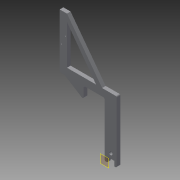
# Autodesk Inventor part: Right Climber Hook
Saved by Autodesk Inventor 2013 (Build 170138000, 138)
## iProperties
Created: 2013-03-16
Part Number: Right Climber Hook
Material: Generic
Document SubType Name: Modeling
Designer: Arpan
Density: 1 g/cm^3
Author: Arpan
Autodesk Inventor part; units mm, degrees
ref_plane "YZ Plane" through (0, 0, 0) normal (1, 0, 0) x (0, 1, 0)
ref_plane "XZ Plane" through (0, 0, 0) normal (0, 1, 0) x (-1, 0, 0)
ref_plane "XY Plane" through (0, 0, 0) normal (0, 0, 1) x (1, 0, 0)
ref_plane "Work Plane1" through (0, 0, 9.525) normal (0, 0, 1) x (1, 0, 0)
sketch "Sketch1" plane through (0, 0, 0) normal (0, 0, 1) x (1, 0, 0)
  line L0 (0, 0) -> (6.35, 0)
  line L1 (6.35, 0) -> (6.35, 12.7)
  line L2 (6.35, 12.7) -> (25.4, 12.7)
  line L3 (25.4, 12.7) -> (25.4, 0)
  line L4 (25.4, 0) -> (31.75, 0)
  line L5 (31.75, 0) -> (31.75, 161.925)
  circle A0 centre (15.875, 25.4) radius 4.7816
  line L6 (-117.475, 161.925) -> (-117.475, 142.875)
  line L7 (0, 142.875) -> (0, 0)
  line L8 (-117.475, 142.875) -> (-117.475, 284.6917)
  line L9 (-54.61, 142.875) -> (-54.61, 111.125)
  line L10 (-54.61, 111.125) -> (-105.41, 142.875)
  line L11 (-117.475, 142.875) -> (-105.41, 142.875)
  line L12 (-54.61, 142.875) -> (0, 142.875)
  line L13 (-98.425, 284.6917) -> (-117.475, 284.6917)
  line L14 (-98.425, 265.5175) -> (-98.425, 256.0855)
  line L15 (-98.425, 238.125) -> (-98.425, 161.925)
  line L16 (31.75, 161.925) -> (-6.4592, 161.925)
  line L17 (-22.225, 161.925) -> (-98.425, 161.925)
  line L18 (-98.425, 284.6917) -> (-6.4592, 161.925)
  line L19 (-22.225, 161.925) -> (-98.425, 265.5175)
  line L20 (-98.425, 238.125) -> (-98.425, 256.0855)
  point P0 (-98.425, 263.525)
  point P1 (-6.35, 161.925)
  dimension "d0" = 6.35
  dimension "d1" = 12.7
  dimension "d2" = 19.05
  dimension "d3" = 6.35
  dimension "d4" = 161.925
  dimension "d5" = 9.5631
  dimension "d6" = 12.7
  dimension "d7" = 9.525
  dimension "d8" = 149.225
  dimension "d9" = 19.05
  dimension "d12" = 54.61
  dimension "d13" = 31.75
  dimension "d14" = 50.8
  dimension "d18" = 127
  dimension "d34" = 122.7667
  dimension "d37" = 19.05
  dimension "d38" = 19.05
  dimension "d39" = 76.2
  dimension "d40" = 76.2
  dimension "d41" = 19.05
  dimension "d50" = 0.5
  dimension "d51" = 12.7
  constraints: 42 end point, 15 perpendicular, 5 parallel, 3 horizontal, 1 centre point, 1 point on line, 1 vertical
  measures "d0" distance of L0.start L0.end
  measures "d1" distance of L0.end L1.end
  measures "d2" distance of L1.end L2.end
  measures "d3" distance of L3.end L4.end
  measures "d4" distance of L4.end L5.end
  measures "d5" diameter of A0
  measures "d6" distance from line of L2 A0.centre
  measures "d7" distance from line of L1 A0.centre
  measures "d8" distance of L5.end L6.start
  measures "d9" distance of L6.start L6.end
  measures "d12" distance between parallel lines of L7 L9
  measures "d13" distance of L9.start L9.end
  measures "d14" distance from line of L9 L10.end
  measures "d18" distance of L17.start point (-98.425, 263.525)
  measures "d34" distance of L15.end L13.start
  measures "d37" distance between parallel lines of L17 L12
  measures "d38" distance between parallel lines of L8 L15
  measures "d39" distance from line of L17 L15.start
  measures "d40" distance from line of L17.start L15
  measures "d41" distance of L13.start L8.end
  measures "d50" angle of L18 L19
  measures "d51" distance from line of L16.end L19
sketch "Sketch2" plane through (0, 0, 9.525) normal (0, 0, 1) x (1, 0, 0)
  line L0 (-98.425, 298.45) -> (-117.475, 298.45) projected
  line L1 (-117.475, 284.6917) -> (-117.475, 142.875) projected
  circle A0 centre (-102.9208, 232.0925) radius 1.5875
  circle A1 centre (-113.03, 209.0801) radius 1.5875
  dimension "d24" = 3.175
  dimension "d25" = 14.5542
  dimension "d26" = 66.3575
  dimension "d27" = 3.175
  dimension "d29" = 89.3699
  dimension "d32" = 4.445
  constraints: 2 centre point
  measures "d24" diameter of A0
  measures "d25" distance from line of L1 A0.centre
  measures "d26" distance from line of A0.centre L0
  measures "d27" diameter of A1
  measures "d29" distance from line of L0 A1.centre
  measures "d32" distance from line of L1 A1.centre
extrude "Extrusion4" add sketch "Sketch1" along normal blind 9.525
extrude "Extrusion5" cut sketch "Sketch2" against normal blind 9.525
fillet "Fillet2" radius 3.175 1 edges at (0, 142.875, 4.7625)
fillet "Fillet3" radius 3.175 1 edges at (-54.61, 142.875, 4.7625)
fillet "Fillet4" radius 3.175 1 edges at (-105.41, 142.875, 4.7625)
fillet "Fillet5" radius 3.175 6 edges at (-117.475, 284.6917, 4.7625) (-98.425, 284.6917, 4.7625) (-6.4592, 161.925, 4.7625) (-22.225, 161.925, 4.7625) (-98.425, 161.925, 4.7625) (-98.425, 265.5175, 4.7625)
sketch "Sketch4" plane through (0, 0, 9.525) normal (0, 0, 1) x (1, 0, 0)
  arc A0 (-97.4725, 283.4202) -> (-100.0136, 284.6917) centre (-100.0136, 281.5167) ccw projected
  line L0 (-100.0136, 284.6917) -> (-114.3, 284.6917) projected
  arc A1 (-114.3, 284.6917) -> (-117.475, 281.5167) centre (-114.3, 281.5167) ccw projected
  line L1 (-117.475, 281.5167) -> (-117.475, 142.875) projected
  line L2 (-117.475, 142.875) -> (-106.3206, 142.875) projected
  arc A2 (-104.6378, 142.3924) -> (-106.3206, 142.875) centre (-106.3206, 139.7) ccw projected
  line L3 (-104.6378, 142.3924) -> (-54.61, 111.125) projected
  line L4 (-54.61, 111.125) -> (-54.61, 139.7) projected
  arc A3 (-51.435, 142.875) -> (-54.61, 139.7) centre (-51.435, 139.7) ccw projected
  line L5 (-51.435, 142.875) -> (-3.175, 142.875) projected
  arc A4 (0, 139.7) -> (-3.175, 142.875) centre (-3.175, 139.7) ccw projected
  line L6 (0, 139.7) -> (0, 0) projected
  line L7 (0, 0) -> (6.35, 0) projected
  line L8 (6.35, 0) -> (6.35, 12.7) projected
  line L9 (6.35, 12.7) -> (25.4, 12.7) projected
  line L10 (25.4, 12.7) -> (25.4, 0) projected
  line L11 (25.4, 0) -> (31.75, 0) projected
  line L12 (31.75, 0) -> (31.75, 161.925) projected
  line L13 (31.75, 161.925) -> (-4.8706, 161.925) projected
  arc A5 (-7.4117, 163.1964) -> (-4.8706, 161.925) centre (-4.8706, 165.1) ccw projected
  line L14 (-7.4117, 163.1964) -> (-97.4725, 283.4202) projected
  line L15 (25.4, 0) -> (38.1, 0)
  line L16 (38.1, 0) -> (38.1, 25.4)
  line L17 (38.1, 25.4) -> (31.75, 25.4)
  dimension "d56" = 12.7
  constraints: 6 end point, 2 perpendicular, 2 point on line
  measures "d56" distance of L10.end L15.end
extrude "Extrusion7" add sketch "Sketch4" against normal blind 9.525 contours L17 L16 L15 L12
fillet "Fillet6" radius 3.175 4 edges at (38.1, 0, 4.7625) (25.4, 0, 4.7625) (6.35, 0, 4.7625) (0, 0, 4.7625)
fillet "Fillet7" radius 6.35 1 edges at (38.1, 25.4, 4.7625)
sketch "Sketch5" plane through (0, 0, 9.525) normal (0, 0, 1) x (1, 0, 0)
  arc A0 (38.1, 19.05) -> (31.75, 25.4) centre (31.75, 19.05) ccw projected
  line L0 (31.75, 25.4) -> (31.75, 161.925) projected
  line L1 (31.75, 161.925) -> (-4.8706, 161.925) projected
  arc A1 (-7.4117, 163.1964) -> (-4.8706, 161.925) centre (-4.8706, 165.1) ccw projected
  line L2 (-7.4117, 163.1964) -> (-97.4725, 283.4202) projected
  arc A2 (-97.4725, 283.4202) -> (-100.0136, 284.6917) centre (-100.0136, 281.5167) ccw projected
  line L3 (-100.0136, 284.6917) -> (-114.3, 284.6917) projected
  arc A3 (-114.3, 284.6917) -> (-117.475, 281.5167) centre (-114.3, 281.5167) ccw projected
  line L4 (-117.475, 281.5167) -> (-117.475, 142.875) projected
  line L5 (-117.475, 142.875) -> (-106.3206, 142.875) projected
  arc A4 (-104.6378, 142.3924) -> (-106.3206, 142.875) centre (-106.3206, 139.7) ccw projected
  line L6 (-104.6378, 142.3924) -> (-54.61, 111.125) projected
  line L7 (-54.61, 111.125) -> (-54.61, 139.7) projected
  arc A5 (-51.435, 142.875) -> (-54.61, 139.7) centre (-51.435, 139.7) ccw projected
  line L8 (-51.435, 142.875) -> (-3.175, 142.875) projected
  arc A6 (0, 139.7) -> (-3.175, 142.875) centre (-3.175, 139.7) ccw projected
  line L9 (0, 139.7) -> (0, 3.175) projected
  arc A7 (0, 3.175) -> (6.35, 3.175) centre (3.175, 3.175) ccw projected
  line L10 (6.35, 3.175) -> (6.35, 12.7) projected
  line L11 (6.35, 12.7) -> (25.4, 12.7) projected
  line L12 (25.4, 12.7) -> (25.4, 3.175) projected
  arc A8 (25.4, 3.175) -> (28.575, 0) centre (28.575, 3.175) ccw projected
  line L13 (28.575, 0) -> (34.925, 0) projected
  arc A9 (34.925, 0) -> (38.1, 3.175) centre (34.925, 3.175) ccw projected
  line L14 (38.1, 3.175) -> (38.1, 19.05) projected
  circle A10 centre (15.875, 25.4) radius 4.7816 projected
  line L15 (-98.425, 165.1) -> (-98.425, 255.8428) projected
  arc A11 (-92.6924, 257.7241) -> (-98.425, 255.8428) centre (-95.25, 255.8428) ccw projected
  line L16 (-92.6924, 257.7241) -> (-25.9443, 166.9813) projected
  arc A12 (-28.5019, 161.925) -> (-25.9443, 166.9813) centre (-28.5019, 165.1) ccw projected
  line L17 (-28.5019, 161.925) -> (-95.25, 161.925) projected
  arc A13 (-98.425, 165.1) -> (-95.25, 161.925) centre (-95.25, 165.1) ccw projected
  circle A14 centre (-113.03, 209.0801) radius 1.5875 projected
  circle A15 centre (-102.9208, 232.0925) radius 1.5875 projected
  point P0 (0, 0)
body "Solid2"
